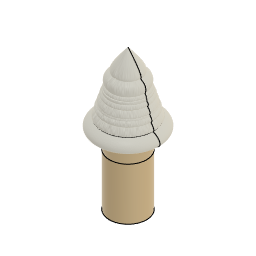
SoftServer v1 (Autodesk Fusion 360 design; units mm, degrees)
Autodesk Fusion 360 part; units mm, degrees
note: some values were not read from the file. Set by a fixed rule: which sketch regions a step uses.
sketch "Sketch1" plane through (0, 0, 0) normal (0, 0, 1) x (1, 0, 0)
  circle A0 centre (0, 0) radius 6.35
  dimension "d1" = 12.7
  constraint coincident A0.centre origin
  measures "d1" diameter of A0
extrude "Extrude1" add sketch "Sketch1" along normal blind 17.78 makes body 1
ref_plane "WorkPlane1" through (0, 0, 25.4) normal (0, 0, 1) x (1, 0, 0)
ref_plane "WorkPlane2" through (0, 0, 25.4) normal (0, 0, 1) x (1, 0, 0)
sketch "Sketch3" plane through (0, 0, 25.4) normal (0, 0, 1) x (1, 0, 0)
  circle A0 centre (0, 0) radius 8.255
  dimension "d7" = 16.51
  constraint coincident A0.centre origin
  measures "d7" diameter of A0
loft "Loft1" add profiles "Sketch3" section 1 face at (0.4605, 1.9232, 17.78) section 2 on bodies 1 bodies 1
sketch "Sketch4" plane through (0, 0, 0) normal (0, 1, 0) x (1, 0, 0)
  line L0 (0.0064, -25.3772) -> (9.6563, -25.3772)
  spline S0 degree 5 poles (9.6563, -25.3772) (9.6408, -25.4423) (9.6082, -25.57) (9.5546, -25.7548) (9.4738, -25.9872) (9.3576, -26.2546) (9.227, -26.4986) (9.0839, -26.7185) (8.9318, -26.9133) (8.7752, -27.0816) (8.6212, -27.2212) (8.4786, -27.3295) (8.3592, -27.4028) (8.277, -27.4372) (8.2432, -27.4325) (8.2634, -27.395) (8.3325, -27.3414) (8.4374, -27.295) (8.5602, -27.2792) (8.6815, -27.3118) (8.7839, -27.4011) (8.8522, -27.5476) (8.8753, -27.7456) (8.8469, -27.9843) (8.7672, -28.2495) (8.6436, -28.5247) (8.4892, -28.7927) (8.3202, -29.0377) (8.1545, -29.2461) (8.0097, -29.4089) (7.9008, -29.523) (7.8386, -29.5924) (7.8276, -29.6309) (7.8643, -29.6622) (7.938, -29.7121) (8.0318, -29.7979) (8.1243, -29.9249) (8.1943, -30.0901) (8.2234, -30.2839) (8.2004, -30.4927) (8.1243, -30.7014) (8.0086, -30.8957) (7.876, -31.0635) (7.7517, -31.1964) (7.658, -31.2915) (7.6077, -31.3525) (7.5982, -31.3912) (7.6052, -31.4293) (7.5979, -31.488) (7.5609, -31.5735) (7.5023, -31.6729) (7.4406, -31.7672) (7.3981, -31.8388) (7.3892, -31.8842) (7.417, -31.9148) (7.4736, -31.9483) (7.5401, -32.0032) (7.5928, -32.095) (7.6096, -32.2336) (7.5769, -32.4193) (7.4934, -32.6417) (7.3663, -32.8839) (7.2094, -33.1256) (7.0408, -33.3462) (6.8801, -33.5286) (6.7465, -33.662) (6.6562, -33.7452) (6.62, -33.791) (6.6407, -33.8221) (6.7106, -33.8625) (6.8084, -33.93) (6.9046, -34.035) (6.9699, -34.1804) (6.9813, -34.3616) (6.9305, -34.5658) (6.8283, -34.7727) (6.697, -34.9599) (6.5646, -35.1075) (6.4574, -35.2035) (6.3945, -35.248) (6.3801, -35.259) (6.3987, -35.2759) (6.4283, -35.333) (6.4534, -35.4368) (6.4639, -35.5749) (6.4542, -35.725) (6.423, -35.8631) (6.3726, -35.9738) (6.3084, -36.0503) (6.2402, -36.0938) (6.1815, -36.1127) (6.1509, -36.1222) (6.1616, -36.1406) (6.2037, -36.1854) (6.2471, -36.269) (6.2591, -36.3959) (6.2198, -36.5582) (6.1337, -36.7347) (6.0195, -36.899) (5.9036, -37.0267) (5.8124, -37.1032) (5.7653, -37.1302) (5.7659, -37.136) (5.8048, -37.1631) (5.8692, -37.241) (5.9459, -37.3825) (6.0212, -37.5881) (6.0823, -37.8489) (6.1177, -38.1494) (6.1182, -38.4713) (6.0778, -38.7956) (5.9945, -39.1066) (5.8708, -39.3938) (5.7125, -39.6509) (5.5282, -39.875) (5.3284, -40.0663) (5.1244, -40.2269) (4.9277, -40.3604) (4.7491, -40.471) (4.5978, -40.5629) (4.4809, -40.6396) (4.4019, -40.7036) (4.3614, -40.7575) (4.3562, -40.8049) (4.3788, -40.8515) (4.4185, -40.9049) (4.4631, -40.9734) (4.5011, -41.0645) (4.5228, -41.1849) (4.5194, -41.3405) (4.4836, -41.5362) (4.409, -41.7763) (4.2901, -42.0644) (4.1225, -42.4035) (3.9025, -42.796) (3.6274, -43.244) (3.2947, -43.7487) (2.903, -44.3115) (2.4509, -44.933) (1.9377, -45.6137) (1.363, -46.3539) (0.8538, -46.9939) (0.4441, -47.5007) (0.1586, -47.8505) (0.0128, -48.0284) knots 0 0 0 0 0 0 0.00714286 0.01428571 0.02142857 0.02857143 0.03571429 0.04285714 0.05 0.05714286 0.06428571 0.07142857 0.07857143 0.08571429 0.09285714 0.1 0.10714286 0.11428571 0.12142857 0.12857143 0.13571429 0.14285714 0.15 0.15714286 0.16428571 0.17142857 0.17857143 0.18571429 0.19285714 0.2 0.20714286 0.21428571 0.22142857 0.22857143 0.23571429 0.24285714 0.25 0.25714286 0.26428571 0.27142857 0.27857143 0.28571429 0.29285714 0.3 0.30714286 0.31428571 0.32142857 0.32857143 0.33571429 0.34285714 0.35 0.35714286 0.36428571 0.37142857 0.37857143 0.38571429 0.39285714 0.4 0.40714286 0.41428571 0.42142857 0.42857143 0.43571429 0.44285714 0.45 0.45714286 0.46428571 0.47142857 0.47857143 0.48571429 0.49285714 0.5 0.50714286 0.51428571 0.52142857 0.52857143 0.53571429 0.54285714 0.55 0.55714286 0.56428571 0.57142857 0.57857143 0.58571429 0.59285714 0.6 0.60714286 0.61428571 0.62142857 0.62857143 0.63571429 0.64285714 0.65 0.65714286 0.66428571 0.67142857 0.67857143 0.68571429 0.69285714 0.7 0.70714286 0.71428571 0.72142857 0.72857143 0.73571429 0.74285714 0.75 0.75714286 0.76428571 0.77142857 0.77857143 0.78571429 0.79285714 0.8 0.80714286 0.81428571 0.82142857 0.82857143 0.83571429 0.84285714 0.85 0.85714286 0.86428571 0.87142857 0.87857143 0.88571429 0.89285714 0.9 0.90714286 0.91428571 0.92142857 0.92857143 0.93571429 0.94285714 0.95 0.95714286 0.96428571 0.97142857 0.97857143 0.98571429 0.99285714 1 1 1 1 1 1
  line L1 (0.0128, -48.0284) -> (0.0064, -25.3772)
  spline S1 degree 5 poles (8.2384, -25.3772) (8.1641, -25.2966) (8.0298, -25.1379) (7.8709, -24.9082) (7.7447, -24.6182) (7.7294, -24.2848) (7.8523, -23.9845) (8.1018, -23.7253) (8.4555, -23.5201) (8.8813, -23.3852) (9.3422, -23.3362) (9.7998, -23.3846) (10.2182, -23.5345) (10.5676, -23.7778) (10.8243, -24.0984) (10.9702, -24.4756) (10.992, -24.888) (10.8815, -25.3176) (10.6347, -25.752) (10.2508, -26.1832) (9.7307, -26.6065) (9.2072, -26.9371) (8.7549, -27.1803) (8.4269, -27.3402) (8.2563, -27.4197) knots 0 0 0 0 0 0 0.05 0.1 0.15 0.2 0.25 0.3 0.35 0.4 0.45 0.5 0.55 0.6 0.65 0.7 0.75 0.8 0.85 0.9 0.95 1 1 1 1 1 1
  point P0 (8.5268, -27.2903)
  point P1 (8.2563, -27.4197)
  point P2 (8.5268, -27.2903)
  point P3 (8.8366, -27.9793)
  point P4 (7.8525, -29.583)
  point P5 (7.9071, -29.6924)
  point P6 (8.1824, -30.5124)
  point P7 (7.6156, -31.3507)
  point P8 (7.5973, -31.4692)
  point P9 (7.4242, -31.7972)
  point P10 (7.4242, -31.9157)
  point P11 (7.5973, -32.189)
  point P12 (6.7226, -33.6834)
  point P13 (6.6588, -33.8292)
  point P14 (6.9686, -34.3303)
  point P15 (6.4094, -35.2376)
  point P16 (6.4006, -35.2842)
  point P17 (6.4446, -35.7485)
  point P18 (6.2325, -36.0927)
  point P19 (6.1605, -36.1328)
  point P20 (6.2485, -36.3729)
  point P21 (5.8042, -37.1054)
  point P22 (5.7842, -37.1494)
  point P23 (6.0818, -38.7096)
  point P24 (4.6676, -40.5208)
  point P25 (4.3625, -40.7824)
  point P26 (4.4352, -40.9325)
  point P27 (7.9512, -23.9055)
  point P28 (9.8358, -23.4209)
  point P29 (10.9665, -24.767)
  constraint horizontal L0
  constraint coincident P2 P0
  constraint coincident L0 S1.start
  constraint coincident P1 S1.end
revolve "Revolve1" add sketch "Sketch4" angle 360 about axis through (0.0128, 0, 48.0284) along (-0.000281, 0, -1) separate body makes body 2
